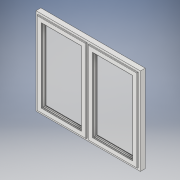
# Autodesk Inventor part: Окно 2 рамы-01
Saved by Autodesk Inventor 2019 (Build 230136000, 136)
## iProperties
Created: 2018-09-18
Part Number: Окно 2 рамы-01
Material: Пластик АБС
Document SubType Name: Modeling
Designer: Андреев Н.Л.
Density: 1.06 g/cm^3
Appearance: Гладкий — белый
ТОЛЩВЫС: 105,000 мм
ДЛИНА: 1800,000 мм
ШИРИНА: 1500,000 мм
ТолщСтекла: 5,000 мм
Author: Андреев Н.Л.
Autodesk Inventor part; units mm, degrees
ref_plane "YZ Plane" through (0, 0, 0) normal (1, 0, 0) x (0, 1, 0)
ref_plane "XZ Plane" through (0, 0, 0) normal (0, 1, 0) x (-1, 0, 0)
ref_plane "XY Plane" through (0, 0, 0) normal (0, 0, 1) x (1, 0, 0)
sketch "Эскиз1" plane through (0, 0, 0) normal (0, 0, 1) x (1, 0, 0)
  line L0 (0, 0) -> (1800, 0) construction
  line L1 (1800, 0) -> (1800, 1500) construction
  line L2 (1800, 1500) -> (0, 1500) construction
  line L3 (0, 1500) -> (0, 0) construction
  line L4 (0, 0) -> (918, 0)
  line L5 (918, 0) -> (918, 1500)
  line L6 (918, 1500) -> (0, 1500)
  line L7 (0, 1500) -> (0, 0)
  dimension "ДЛИНА" = 1800
  dimension "ШИРИНА" = 1500
  dimension "d15" = 918
  constraints: 16 end point, 4 parallel, 2 horizontal, 2 perpendicular, 1 point on line
  measures "ДЛИНА" distance of L2.end L1.end
  measures "ШИРИНА" distance of L1.end L0.end
  measures "d15" distance between parallel lines of L7 L5
sketch "Эскиз2" plane through (0, 0, 0) normal (0, 1, 0) x (-1, 0, 0)
  line L0 (0, -84) -> (0, 0)
  line L1 (0, -84) -> (-61.2196, -84)
  arc A0 (-65.918, -80.7101) -> (-61.2196, -84) centre (-61.2196, -79) ccw
  line L2 (-65.918, -80.7101) -> (-72, -64)
  line L3 (-72, -64) -> (-45, -64)
  line L4 (-45, -64) -> (-45, 0)
  line L5 (-45, 0) -> (0, 0)
  line L6 (-63.5599, -64) -> (-108.4522, -64)
  arc A1 (-116.3916, -58.3251) -> (-108.4522, -64) centre (-108.4522, -55.6088) ccw
  line L7 (-116.3916, -58.3251) -> (-120, -47.7784)
  line L8 (-120, -47.7784) -> (-120, -43.4944)
  line L9 (-120, -43.4944) -> (-99.8724, -43.4944)
  line L10 (-99.8724, -43.4944) -> (-99.8724, 4.5056)
  line L11 (-99.8724, 4.5056) -> (-120, 4.5056)
  line L12 (-120, 4.5056) -> (-120, 7.7024)
  line L13 (-120, 7.7024) -> (-117.378, 17.0929)
  arc A2 (-112.2629, 21) -> (-117.378, 17.0929) centre (-112.2629, 15.6982) ccw
  line L14 (-112.2629, 21) -> (-42.9824, 21)
  arc A3 (-36, 14.0176) -> (-42.9824, 21) centre (-42.9824, 14.0176) ccw
  line L15 (-36, 14.0176) -> (-36, 0)
  line L16 (-36, 0) -> (-58.0741, 0)
  line L17 (-58.0741, 0) -> (-58.0741, -40.9171)
  line L18 (-58.0741, -40.9171) -> (-63.5599, -40.9171)
  line L19 (-63.5599, -40.9171) -> (-63.5599, -64)
  point P0 (0, 0)
  dimension "d2" = 84
  dimension "d3" = 72
  dimension "d4" = 5
  dimension "d5" = 110
  dimension "d6" = 20
  dimension "d7" = 45
  dimension "d8" = 120
  dimension "d9" = 48
  dimension "d10" = 36
  dimension "ТОЛЩВЫС" = 105
  constraints: 40 end point, 10 perpendicular, 8 point on circle, 7 tangent, 4 centre point, 2 collinear, 2 point on line
  measures "d2" distance of L0.start L0.end
  measures "d3" distance from line of L0 L2.end
  measures "d4" radius of A0
  measures "d5" angle of L1 L2
  measures "d6" distance between parallel lines of L3 L1
  measures "d7" distance between parallel lines of L0 L4
  measures "d8" distance between parallel lines of L8 L0
  measures "d9" distance between parallel lines of L11 L9
  measures "d10" distance between parallel lines of L15 L0
  measures "ТОЛЩВЫС" distance between parallel lines of L1 L14
sweep "Сдвиг1" add profiles "Эскиз2" path "Эскиз1" path curves L7 L6 L5 L4 contours L1 A0 L2 L3 L4 L5 L0
pattern_linear "Прямоуг.массив1" count 2 spacing 882 along (1, 0, 0)
sweep "Сдвиг2" add profiles "Эскиз2" path "Эскиз1" separate body path curves L7 L6 L5 L4 contours L5 L16 L17 L18 L19 L3 L6 A1 L7 L8 L9 L10 L11 L12 L13 A2 L14 A3 L15
sketch "Эскиз3" plane through (99.8724, 99.8724, -43.4944) normal (0, 1, 0) x (1, 0, 0)
  line L0 (718.2552, -48) -> (718.2552, 0) construction
  line L1 (718.2552, 0) -> (0, 0) construction
  line L2 (0, -48) -> (0, 0) construction
  line L3 (718.2552, -48) -> (0, -48) construction
  line L4 (718.2552, -48) -> (718.2552, 0) projected
  line L5 (0, 0) -> (718.2552, 0)
  line L6 (718.2552, 0) -> (718.2552, -5)
  line L7 (718.2552, -5) -> (0, -5)
  line L8 (0, -5) -> (0, 0)
  point P0 (-99.8724, -43.4944)
  dimension "ТолщСтекла" = 5
  constraints: 8 end point, 2 parallel, 1 horizontal, 1 perpendicular, 1 point on line
  measures "ТолщСтекла" distance of L5.end L6.end
extrude "Выдавливание1" add sketch "Эскиз3" along normal up to surface (1300.2552 mm away) separate body
pattern_linear "Прямоуг.массив2" count 3 spacing 21.5 along (0, 0, 1) count 2 spacing 882 along (1, 0, 0) of "Выдавливание1" bodies 3
pattern_linear "Прямоуг.массив3" count 2 spacing 882 along (1, 0, 0) of "Сдвиг2" bodies 2
